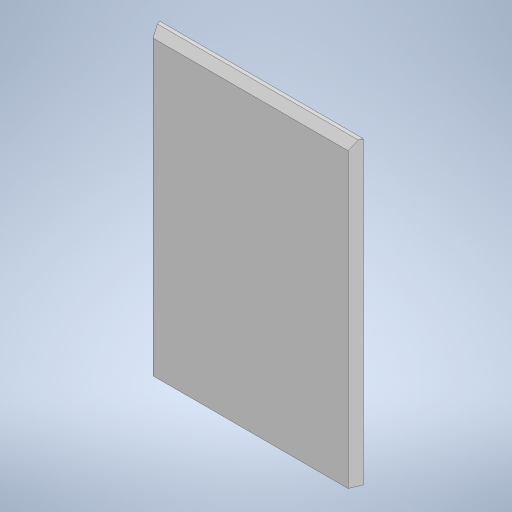
# Autodesk Inventor part: PotiBoxLid
Saved by Autodesk Inventor 2024.3 (Build 283343000, 343)
## iProperties
Created: 2025-03-30
Part Number: PotiBoxLid
Material: Generisch
Document SubType Name: Modeling
Designer: maxho
Density: 1 g/cm^3
Appearance: Vorgabe
Author: maxho
## iProperties of the stored document PotiBoxLid_3D-Druck.ipt
Created: 2025-03-30
Part Number: PotiBoxLid_3D-Druck
Material: Generisch
Document SubType Name: Modeling
Designer: maxho
Density: 1 g/cm^3
Appearance: Vorgabe
Author: maxho
Autodesk Inventor part; units mm, degrees
ref_plane "YZ Plane" through (0, 0, 0) normal (1, 0, 0) x (0, 1, 0)
ref_plane "XZ Plane" through (0, 0, 0) normal (0, 1, 0) x (-1, 0, 0)
ref_plane "XY Plane" through (0, 0, 0) normal (0, 0, 1) x (1, 0, 0)
sketch "Skizze1" plane through (0, 0, 0) normal (0, 0, 1) x (1, 0, 0)
  line L0 (0, 0) -> (-1.2426, 3)
  line L1 (-1.2426, 3) -> (55.2426, 3)
  line L2 (55.2426, 3) -> (54, 0)
  line L3 (54, 0) -> (0, 0)
  point P0 (27, 3)
  point P1 (27, 0)
  dimension "d1" = 112.5
  dimension "d2" = 3
  dimension "d3" = 54
  constraints: 8 end point, 2 midpoint, 1 horizontal, 1 parallel, 1 vertical alignment
  measures "d1" angle of L3 L0
  measures "d2" distance between parallel lines of L1 L3
  measures "d3" distance of L2.end L0.start
extrude "Extrusion1" add sketch "Skizze1" along normal blind 83
chamfer "Fasen1" distance 2 angle 45 1 edges at (27, 0, 83)
sketch "Skizze2" plane through (0, 0, 0) normal (0, -1, 0) x (1, 0, 0)
  line L0 (0, 81) -> (54, 81) projected
  line L1 (0, 0) -> (0, 81) projected
  line L2 (0, 0) -> (54, 0) projected
  line L3 (54, 0) -> (54, 81) projected
  line L4 (57, 81) -> (-3, 81)
  line L5 (-3, 81) -> (-1, 83)
  line L6 (-1, 83) -> (55, 83)
  line L7 (55.2426, 83) -> (-1.2426, 83) projected
  line L8 (55, 83) -> (57, 81)
  line L9 (0, 81) -> (54, 81) projected
  line L10 (-1.2426, 0) -> (-1.2426, 83) projected
  line L11 (55.2426, 0) -> (55.2426, 83) projected
  point P0 (27, 81)
  point P1 (27, 81)
  point P2 (27, 83)
  point P3 (-1.2426, 82.7574)
  point P4 (55.2426, 82.7574)
  dimension "d9" = 60
  dimension "d10" = 45
  constraints: 8 end point, 5 midpoint, 1 collinear, 1 horizontal, 1 vertical alignment
  measures "d9" distance of L4.start L4.end
  measures "d10" angle of L4 L8
extrude "Extrusion2" cut sketch "Skizze2" against normal through all contours L10 L7 L5 | L8 L7 L11
equation "\"d2\" = PotiBoxThickness"
equation "\"d3\" = PotiBoxInnerWidth"
equation "\"d4\" = PotiBoxInnerLength + PotiBoxThickness"
equation "\"d9\" = PotiBoxInnerWidth + 2 * PotiBoxThickness"
equation "\"PotiBoxThickness\" = 3"
equation "\"PotiBoxInnerWidth\" = 54"
equation "\"PotiBoxInnerLength\" = 80"
